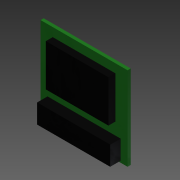
# Autodesk Inventor part: RasCam
Saved by Autodesk Inventor 2014 SP1 (Build 180222100, 222)
## iProperties
Created: 2014-02-08
Part Number: RasCam
Material: Generic
Document SubType Name: Modeling
Designer: Jack
Density: 1 g/cm^3
Appearance: Smooth - Black
Author: Jack
Autodesk Inventor part; units mm, degrees
ref_plane "YZ Plane" through (0, 0, 0) normal (1, 0, 0) x (0, 1, 0)
ref_plane "XZ Plane" through (0, 0, 0) normal (0, 1, 0) x (-1, 0, 0)
ref_plane "XY Plane" through (0, 0, 0) normal (0, 0, 1) x (1, 0, 0)
sketch "Sketch1" plane through (0, 0, 0) normal (0, 1, 0) x (-1, 0, 0)
  line L0 (0, 0) -> (25, 0)
  line L1 (25, 0) -> (25, 24)
  line L2 (25, 24) -> (0, 24)
  line L3 (0, 24) -> (0, 0)
  dimension "d0" = 25
  dimension "d1" = 24
  constraints: 8 end point, 3 perpendicular, 1 horizontal
  measures "d0" distance of L0.start L0.end
  measures "d1" distance of L0.end L1.end
extrude "Extrusion1" add sketch "Sketch1" along normal blind 0.9
sketch "Sketch2" plane through (0, 0, 0) normal (0, -1, 0) x (1, 0, 0)
  line L0 (0, 24) -> (0, 0) projected
  line L1 (-25, 24) -> (0, 24) projected
  line L2 (-3.5, 9.5) -> (-21.5, 9.5)
  line L3 (-21.5, 9.5) -> (-21.5, 21.5)
  line L4 (-21.5, 21.5) -> (-3.5, 21.5)
  line L5 (-3.5, 21.5) -> (-3.5, 9.5)
  dimension "d4" = 12
  dimension "d5" = 18
  dimension "d6" = 3.5
  dimension "d7" = 2.5
  constraints: 8 end point, 2 parallel, 1 horizontal, 1 perpendicular
  measures "d4" distance of L4.end L2.start
  measures "d5" distance of L2.start L2.end
  measures "d6" distance between parallel lines of L0 L5
  measures "d7" distance between parallel lines of L1 L4
extrude "Extrusion2" add sketch "Sketch2" along normal blind 2
sketch "Sketch3" plane through (0, 0.9, 0) normal (0, 1, 0) x (1, 0, 0)
  line L0 (0, 0) -> (-25, 0) projected
  line L1 (0, -24) -> (0, 0) projected
  line L2 (-16.5, -5.5) -> (-8.5, -5.5)
  line L3 (-8.5, -5.5) -> (-8.5, -13.5)
  line L4 (-8.5, -13.5) -> (-16.5, -13.5)
  line L5 (-16.5, -13.5) -> (-16.5, -5.5)
  dimension "d10" = 8
  dimension "d11" = 8
  dimension "d12" = 8.5
  dimension "d13" = 5.5
  constraints: 8 end point, 2 parallel, 1 horizontal, 1 perpendicular
  measures "d10" distance of L2.start L2.end
  measures "d11" distance of L4.end L2.start
  measures "d12" distance between parallel lines of L1 L3
  measures "d13" distance between parallel lines of L0 L2
extrude "Extrusion3" add sketch "Sketch3" along normal blind 4
sketch "Sketch4" plane through (0, 4.9, 0) normal (0, 1, 0) x (1, 0, 0)
  line L0 (-8.5, -5.5) -> (-16.5, -5.5) projected
  line L1 (-8.5, -13.5) -> (-8.5, -5.5) projected
  circle A0 centre (-12.5, -9.5) radius 3.75
  point P0 (0, 0)
  dimension "d16" = 7.5
  dimension "d17" = 4
  dimension "d18" = 4
  constraints: 1 centre point
  measures "d16" diameter of A0
  measures "d17" distance from line of L0 A0.centre
  measures "d18" distance from line of L1 A0.centre
extrude "Extrusion4" add sketch "Sketch4" along normal blind 1.5
sketch "Sketch5" plane through (0, 0.9, 0) normal (0, 1, 0) x (1, 0, 0)
  line L0 (-8.5, -13.5) -> (-16.5, -13.5) projected
  line L1 (-16.5, -13.5) -> (-16.5, -5.5) projected
  line L2 (0, -24) -> (0, 0) projected
  line L3 (-16.25, -22.5) -> (-8.75, -22.5)
  line L4 (-8.75, -22.5) -> (-8.75, -17.5)
  line L5 (-16.25, -17.5) -> (-16.25, -22.5)
  line L6 (-9.75, -17.5) -> (-9.75, -13.5)
  line L7 (-15.25, -17.5) -> (-15.25, -13.5)
  line L8 (-8.75, -17.5) -> (-9.75, -17.5)
  line L9 (-15.25, -17.5) -> (-16.25, -17.5)
  dimension "d21" = 7.5
  dimension "d22" = 5
  dimension "d24" = 0.25
  dimension "d25" = 1
  dimension "d26" = 1
  dimension "d27" = 4
  dimension "d28" = 4
  constraints: 14 end point, 5 perpendicular, 2 parallel, 2 point on line
  measures "d21" distance of L3.start L3.end
  measures "d22" distance of L3.end L4.end
  measures "d24" distance between parallel lines of L1 L5
  measures "d25" distance between parallel lines of L5 L7
  measures "d26" distance between parallel lines of L4 L6
  measures "d27" distance between parallel lines of L0 L9
  measures "d28" distance between parallel lines of L0 L8
extrude "Extrusion5" add sketch "Sketch5" along normal blind 1.5
sketch "Sketch6" plane through (0, 0.9, 0) normal (0, 1, 0) x (1, 0, 0)
  line L0 (-25, 0) -> (-25, -24) projected
  line L1 (-25, -24) -> (0, -24) projected
  circle A0 centre (-20, -19) radius 1
  dimension "d31" = 2
  dimension "d32" = 5
  dimension "d33" = 5
  constraints: 1 centre point
  measures "d31" diameter of A0
  measures "d32" distance from line of L1 A0.centre
  measures "d33" distance from line of L0 A0.centre
extrude "Extrusion6" add sketch "Sketch6" along normal blind 0.5
sketch "Sketch7" plane through (0, 0, 0) normal (0, -1, 0) x (1, 0, 0)
  line L0 (0, 0) -> (-25, 0) projected
  line L1 (-25, 0) -> (-25, 24) projected
  line L2 (-23, 6) -> (-2, 6)
  line L3 (-2, 6) -> (-2, 0.5)
  line L4 (-2, 0.5) -> (-23, 0.5)
  line L5 (-23, 0.5) -> (-23, 6)
  dimension "d36" = 21
  dimension "d37" = 5.5
  dimension "d38" = 2
  dimension "d39" = 0.5
  constraints: 8 end point, 3 perpendicular, 1 parallel
  measures "d36" distance of L2.start L2.end
  measures "d37" distance of L2.end L3.end
  measures "d38" distance between parallel lines of L1 L5
  measures "d39" distance between parallel lines of L0 L4
extrude "Extrusion7" add sketch "Sketch7" along normal blind 3
body "Solid1"
